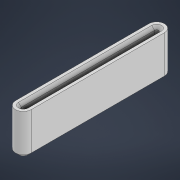
# Autodesk Inventor part: pin_header_protector
Saved by Autodesk Inventor 2022 (Build 260153000, 153)
## iProperties
Created: 2023-02-02
Part Number: pin_header_protector
Material: Generic
Document SubType Name: Modeling
Designer: erwin
Density: 1 g/cm^3
Appearance: Default
Author: erwin
Autodesk Inventor part; units mm, degrees
ref_plane "YZ Plane" through (0, 0, 0) normal (1, 0, 0) x (0, 1, 0)
ref_plane "XZ Plane" through (0, 0, 0) normal (0, 1, 0) x (-1, 0, 0)
ref_plane "XY Plane" through (0, 0, 0) normal (0, 0, 1) x (1, 0, 0)
sketch "Sketch1" plane through (0, 0, 0) normal (0, 1, 0) x (-1, 0, 0)
  line L0 (-1.35, 11.55) -> (-1.35, -11.55)
  line L1 (1.35, -11.55) -> (1.35, 11.55)
  arc A0 (1.35, 11.55) -> (-1.35, 11.55) centre (0, 11.55) ccw
  arc A1 (-1.35, -11.55) -> (1.35, -11.55) centre (0, -11.55) ccw
  line L2 (0, 12.9) -> (0, -12.9) construction
  point P0 (0, 0)
  point P1 (0, 0)
  dimension "d0" = 2.7
  dimension "d2" = 25.8
  constraints: 6 end point, 6 point on circle, 4 tangent, 2 centre point, 1 coincident, 1 midpoint, 1 parallel
  measures "d0" distance between parallel lines of L1 L0
  measures "d2" distance of L2.start L2.end
extrude "Extrusion1" add sketch "Sketch1" along normal blind 7
sketch "Sketch2" plane through (0, 7, 0) normal (0, 1, 0) x (1, 0, 0)
  line L0 (0.35, -11.55) -> (0.35, 11.55)
  line L1 (-0.35, 11.55) -> (-0.35, -11.55)
  arc A0 (-0.35, -11.55) -> (0.35, -11.55) centre (0, -11.55) ccw
  arc A1 (0.35, 11.55) -> (-0.35, 11.55) centre (0, 11.55) ccw
  line L2 (0, -11.9) -> (0, 11.9) construction
  point P0 (0, 0)
  point P1 (0, 0)
  dimension "d5" = 23.8
  dimension "d6" = 0.7
  constraints: 6 end point, 6 point on circle, 4 tangent, 2 centre point, 1 coincident, 1 midpoint, 1 parallel
  measures "d5" distance of L2.start L2.end
  measures "d6" distance between parallel lines of L0 L1
extrude "Extrusion2" cut sketch "Sketch2" against normal blind 6
chamfer "Chamfer1" distance 0.5 angle 45 4 edges at (1.35, 0, 0) (0, 0, -12.9) (-1.35, 0, 0) (0, 0, 12.9)
chamfer "Chamfer2" distance 0.5 angle 45 4 edges at (-0.35, 7, 0) (0, 7, -11.9) (0.35, 7, 0) (0, 7, 11.9)
equation "\"d5\" = pinlength"
equation "\"d6\" = pinwidth"
equation "\"d7\" = pinheight"
equation "\"pinwidth\" = 0.7"
equation "\"pinheight\" = 6"
equation "\"pinlength\" = 23.8"
body "Solid1"
